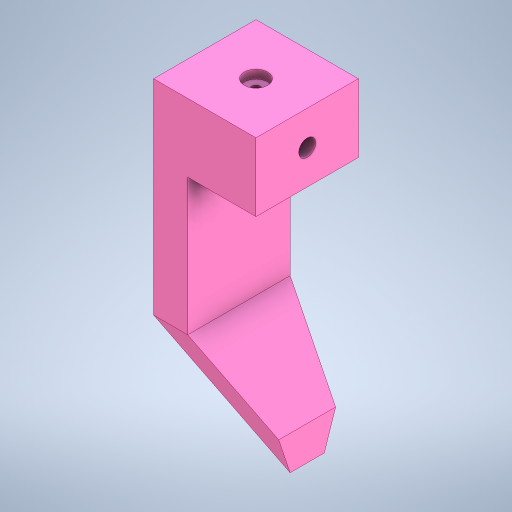
# Autodesk Inventor part: Claw_Finger_BR
Saved by Autodesk Inventor 2024 (Build 280153000, 153)
## iProperties
Created: 2023-10-06
Part Number: Claw_Finger_BR
Material: PET Plastic
Document SubType Name: Modeling
Designer: tangl
Density: 1.541 g/cm^3
Appearance: Pink
Author: tangl
Autodesk Inventor part; units mm, degrees
ref_plane "YZ Plane" through (0, 0, 0) normal (1, 0, 0) x (0, 1, 0)
ref_plane "XZ Plane" through (0, 0, 0) normal (0, 1, 0) x (-1, 0, 0)
ref_plane "XY Plane" through (0, 0, 0) normal (0, 0, 1) x (1, 0, 0)
sketch "Sketch1" plane through (0, 0, 0) normal (0, 0, 1) x (1, 0, 0)
  line L0 (0, 0) -> (-28.5267, 28.5267) construction
  line L1 (-28.5267, 28.5267) -> (-79.3267, 28.5267)
  line L2 (-79.3267, -73.0733) -> (-28.5267, -123.8733)
  line L3 (-28.5267, -123.8733) -> (-28.5267, -149.2733)
  line L4 (-28.5267, -149.2733) -> (-104.7267, -73.0733)
  line L5 (-104.7267, -73.0733) -> (-104.7267, 79.3267)
  line L6 (-79.3267, -73.0733) -> (-79.3267, 28.5267)
  line L7 (-28.5267, 28.5267) -> (-28.5267, 79.3267)
  line L8 (-28.5267, 79.3267) -> (-104.7267, 79.3267)
  point P0 (-28.5267, 153.9136)
  dimension "d11" = 101.6
  dimension "d12" = 50.8
  dimension "d13" = 25.4
  dimension "d17" = 28.5267
  dimension "d18" = 50.8
  dimension "d23" = 135
  dimension "d24" = 17.9605
  dimension "d25" = 50.8
  dimension "d26" = 152.4
  constraints: 18 end point, 3 parallel, 2 vertical, 1 horizontal, 1 perpendicular, 1 point on line
  measures "d11" distance of L1.end L2.start
  measures "d12" horizontal distance of L2.start L2.end
  measures "d13" distance of L2.end L3.end
  measures "d17" horizontal distance of L0.start L0.end
  measures "d18" distance of L0.end L1.end
  measures "d23" angle of L2 L6
  measures "d24" distance between parallel lines of L4 L2
  measures "d25" distance of L0.end L7.end
  measures "d26" distance of L4.end L5.end
extrude "Extrusion1" add sketch "Sketch1" along normal blind 76.2
ref_plane "Work Plane1" through (-155.5267, -73.0733, 0) normal (-1, 0, 0) x (0, 0, 1)
sketch "Sketch2" plane through (-155.5267, -73.0733, 0) normal (-1, 0, 0) x (0, 0, 1)
  line L0 (0, -76.2) -> (76.2, -76.2) projected
  line L1 (76.2, -76.2) -> (50.8, -76.2)
  line L2 (76.2, 0) -> (76.2, 101.6) projected
  line L3 (50.8, -76.2) -> (76.2, 0)
  line L4 (76.2, 0) -> (76.2, -76.2)
  line L5 (0, 0) -> (0, -76.2) projected
  line L6 (0, -76.2) -> (25.4, -76.2)
  line L7 (25.4, -76.2) -> (0, 0)
  line L8 (0, 0) -> (0, -76.2)
  point P0 (0, 73.0733)
  dimension "d28" = 25.4
  dimension "d29" = 25.4
  constraints: 12 end point, 2 collinear, 2 point on line
  measures "d28" distance of L0.end L1.end
  measures "d29" distance of L0.start L6.end
extrude "Extrusion2" cut sketch "Sketch2" against normal blind 177.8
sketch "Sketch3" plane through (-104.7267, 79.3267, 0) normal (0, 1, 0) x (1, 0, 0)
  circle A0 centre (38.1, -38.1) radius 8.7376
  line L0 (76.2, 0) -> (0, 0) projected
  line L1 (76.2, 0) -> (76.2, -76.2) projected
  point P0 (104.7267, 0)
  dimension "d32" = 38.1
  dimension "d33" = 38.1
  dimension "d34" = 17.4752
  constraints: 1 centre point
  measures "d32" distance from line of L0 A0.centre
  measures "d33" distance from line of L1 A0.centre
  measures "d34" diameter of A0
extrude "Extrusion3" cut sketch "Sketch3" against normal blind 6.35
sketch "Sketch4" plane through (-28.5267, 28.5267, 0) normal (1, 0, 0) x (0, 0, -1)
  circle A0 centre (-38.1, 25.4) radius 6.35
  line L0 (0, 0) -> (0, 50.8) projected
  line L1 (0, 0) -> (-76.2, 0) projected
  point P0 (0, -28.5267)
  point P1 (-38.1, 0)
  dimension "d39" = 12.7
  dimension "d40" = 38.1
  dimension "d41" = 25.4
  constraints: 1 centre point, 1 midpoint
  measures "d39" diameter of A0
  measures "d40" distance from line of L0 A0.centre
  measures "d41" distance of point (-38.1, 0) A0.centre
extrude "Extrusion4" cut sketch "Sketch4" against normal blind 153.9875
sketch "Sketch5" plane through (-66.6267, 72.9767, 38.1) normal (0, 1, 0) x (1, 0, 0)
  circle A0 centre (0, 0) radius 3.175
  point P0 (66.6267, 38.1)
  dimension "d44" = 6.35
  constraints: 1 centre point
  measures "d44" diameter of A0
extrude "Extrusion5" cut sketch "Sketch5" against normal blind 3.175
body "Solid1"
